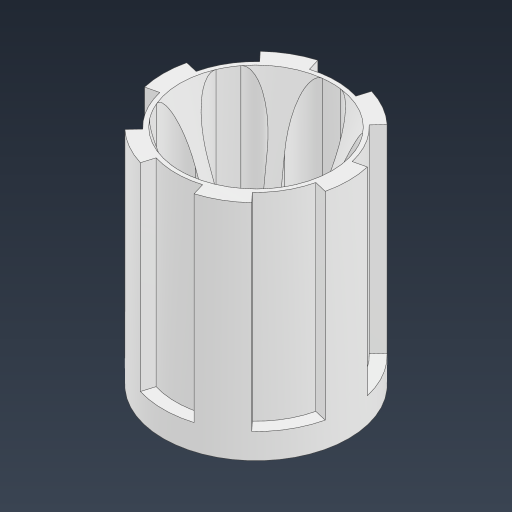
# Autodesk Inventor part: felga
Saved by Autodesk Inventor 2023 (Build 270158000, 158)
## iProperties
Created: 2024-06-08
Part Number: felga
Material: ABS Plastic
Document SubType Name: Modeling
Designer: szymo
Density: 1.06 g/cm^3
Appearance: Smooth - White
Mass: 25.2553 g
Surface Area: 202.96 cm^2
Volume: 23.8257 cm^3
Author: szymo
Autodesk Inventor part; units mm, degrees
ref_plane "YZ Plane" through (0, 0, 0) normal (1, 0, 0) x (0, 1, 0)
ref_plane "XZ Plane" through (0, 0, 0) normal (0, 1, 0) x (-1, 0, 0)
ref_plane "XY Plane" through (0, 0, 0) normal (0, 0, 1) x (1, 0, 0)
sketch "Sketch1" plane through (0, 0, 0) normal (0, 1, 0) x (-1, 0, 0)
  circle A0 centre (0, 0) radius 25
  circle A1 centre (0, 0) radius 22
  circle A2 centre (0, 0) radius 18
  dimension "d0" = 50
  dimension "d1" = 3
  dimension "d2" = 4
  constraints: 3 centre point, 3 coincident
  measures "d0" diameter of A0
  measures "d1" radial gap between concentric circles of A0 A1
  measures "d2" radial gap between concentric circles of A1 A2
extrude "Extrusion1" add sketch "Sketch1" along normal blind 53 contours A1
sketch "Sketch2" plane through (0, 0, 0) normal (0, 1, 0) x (-1, 0, 0)
  circle A0 centre (0, 0) radius 22 projected
  circle A1 centre (0, 0) radius 18 projected
  circle A2 centre (0, 0) radius 5
  line L0 (0, 0) -> (18, 0) construction
  circle A3 centre (0, 0) radius 18 projected
  line L1 (4.7697, 1.5) -> (17.9374, 1.5)
  line L2 (17.9374, -1.5) -> (4.7697, -1.5)
  line L3 (1.0858, 4.8807) -> (7.6697, 16.2842)
  line L4 (0, 0) -> (9, 15.5885) construction
  line L5 (10.2677, 14.7842) -> (3.6839, 3.3807)
  line L6 (-3.6839, 3.3807) -> (-10.2677, 14.7842)
  line L7 (0, 0) -> (-9, 15.5885) construction
  line L8 (-7.6697, 16.2842) -> (-1.0858, 4.8807)
  line L9 (-4.7697, -1.5) -> (-17.9374, -1.5)
  line L10 (0, 0) -> (-18, 0) construction
  line L11 (-17.9374, 1.5) -> (-4.7697, 1.5)
  line L12 (-1.0858, -4.8807) -> (-7.6697, -16.2842)
  line L13 (0, 0) -> (-9, -15.5885) construction
  line L14 (-10.2677, -14.7842) -> (-3.6839, -3.3807)
  line L15 (3.6839, -3.3807) -> (10.2677, -14.7842)
  line L16 (0, 0) -> (9, -15.5885) construction
  line L17 (7.6697, -16.2842) -> (1.0858, -4.8807)
  point P0 (3.6839, 3.3807)
  point P1 (10.2677, 14.7842)
  point P2 (7.6697, 16.2842)
  point P3 (1.0858, 4.8807)
  point P4 (-1.0858, 4.8807)
  point P5 (-7.6697, 16.2842)
  point P6 (-3.6839, 3.3807)
  point P7 (-4.7697, 1.5)
  point P8 (-17.9374, 1.5)
  point P9 (-4.7697, -1.5)
  point P10 (-3.6839, -3.3807)
  point P11 (-10.2677, -14.7842)
  point P12 (-7.6697, -16.2842)
  point P13 (-1.0858, -4.8807)
  point P14 (1.0858, -4.8807)
  point P15 (10.2677, -14.7842)
  point P16 (3.6839, -3.3807)
  dimension "d5" = 10
  dimension "d6" = 1.5
  dimension "d7" = 1.5
  dimension "d10" = 360
  constraints: 36 end point, 5 point on circle, 2 parallel, 1 centre point, 1 coincident, 1 horizontal, 55 other
  measures "d5" diameter of A2
  measures "d6" distance between parallel lines of L1 L0
  measures "d7" distance between parallel lines of L0 L2
extrude "Extrusion2" add sketch "Sketch2" along normal blind 17 contours A1 L2 A2 L1 | L5 A2 L3 A1 | A2 | A1 L17 A2 L15 | L8 A2 L6 A1 | A1 L14 A2 L12 | L11 A2 L9 A1
chamfer "Chamfer1" distance 36 distance2 13 7 edges at (9, 17, 15.5885) (18, 17, 0) (9, 17, -15.5885) (-9, 17, -15.5885) (-17.9843, 17, 0.7507) (-17.9843, 17, -0.7507) (-9, 17, 15.5885) measured on face at (-17.9843, 17.5, 0.7507) measured on face at (-9, 17.5, 15.5885) measured on face at (9, 17.5, 15.5885) measured on face at (-17.9843, 17.5, -0.7507) measured on face at (18, 17.5, 0) measured on face at (9, 17.5, -15.5885) measured on face at (-9, 17.5, -15.5885)
sketch "Sketch3" plane through (0, 0, 0) normal (0, -1, 0) x (1, 0, 0)
  circle A0 centre (0, 0) radius 3
  line L0 (-1.9261, 2.3) -> (1.9261, 2.3)
  line L1 (1.9261, -2.3) -> (-1.9261, -2.3)
  dimension "d19" = 6
  dimension "d20" = 4.6
  dimension "d21" = 2.3
  dimension "d22" = 2.3
  constraints: 4 end point, 4 point on circle, 1 centre point, 1 coincident, 1 horizontal, 1 parallel
  measures "d19" diameter of A0
  measures "d20" distance between parallel lines of L0 L1
  measures "d21" distance from line of L0 point (0, 0)
  measures "d22" distance from line of L1 point (0, 0)
extrude "Extrusion3" cut sketch "Sketch3" against normal blind 12 contours A0 L1 L0
sketch "Sketch6" plane through (0, 0, 0) normal (0, -1, 0) x (1, 0, 0)
  circle A0 centre (0, 0) radius 22 projected
  circle A1 centre (0, -10) radius 3.5
  arc A2 (-7.6697, -16.2842) -> (7.6697, -16.2842) centre (0, 0) ccw projected
  arc A3 (-7.6697, -16.2842) -> (7.6697, -16.2842) centre (0, 0) ccw projected
  circle A4 centre (0, -14.8667) radius 3.1333
  circle A5 centre (12.8749, -7.4333) radius 3.1333
  circle A6 centre (8.6603, -5) radius 3.5
  circle A7 centre (12.8749, 7.4333) radius 3.1333
  circle A8 centre (8.6603, 5) radius 3.5
  circle A9 centre (0, 14.8667) radius 3.1333
  circle A10 centre (0, 10) radius 3.5
  circle A11 centre (-12.8749, 7.4333) radius 3.1333
  circle A12 centre (-8.6603, 5) radius 3.5
  circle A13 centre (-12.8749, -7.4333) radius 3.1333
  circle A14 centre (-8.6603, -5) radius 3.5
  line L0 (-1.0858, -4.8807) -> (-7.6697, -16.2842) projected
  arc A15 (-1.0858, -4.8807) -> (1.0858, -4.8807) centre (0, 0) ccw projected
  line L1 (7.6697, -16.2842) -> (1.0858, -4.8807) projected
  arc A16 (1.0858, 4.8807) -> (-1.0858, 4.8807) centre (0, 0) ccw projected
  arc A17 (4.7697, 1.5) -> (3.6839, 3.3807) centre (0, 0) ccw projected
  arc A18 (3.6839, -3.3807) -> (4.7697, -1.5) centre (0, 0) ccw projected
  arc A19 (-1.0858, -4.8807) -> (1.0858, -4.8807) centre (0, 0) ccw projected
  arc A20 (-4.7697, -1.5) -> (-3.6839, -3.3807) centre (0, 0) ccw projected
  arc A21 (-3.6839, 3.3807) -> (-4.7697, 1.5) centre (0, 0) ccw projected
  line L2 (-1.9261, 2.3) -> (1.9261, 2.3) projected
  arc A22 (1.9261, -2.3) -> (1.9261, 2.3) centre (0, 0) ccw projected
  line L3 (1.9261, -2.3) -> (-1.9261, -2.3) projected
  arc A23 (-1.9261, 2.3) -> (-1.9261, -2.3) centre (0, 0) ccw projected
  arc A24 (-7.6697, -16.2842) -> (7.6697, -16.2842) centre (0, 0) ccw projected
  line L4 (-1.0858, -4.8807) -> (-7.6697, -16.2842) projected
  arc A25 (-1.0858, -4.8807) -> (1.0858, -4.8807) centre (0, 0) ccw projected
  line L5 (7.6697, -16.2842) -> (1.0858, -4.8807) projected
  line L6 (3.6839, -3.3807) -> (10.2677, -14.7842) projected
  arc A26 (3.6839, -3.3807) -> (4.7697, -1.5) centre (0, 0) ccw projected
  line L7 (17.9374, -1.5) -> (4.7697, -1.5) projected
  arc A27 (10.2677, -14.7842) -> (17.9374, -1.5) centre (0, 0) ccw projected
  line L8 (4.7697, 1.5) -> (17.9374, 1.5) projected
  arc A28 (4.7697, 1.5) -> (3.6839, 3.3807) centre (0, 0) ccw projected
  line L9 (10.2677, 14.7842) -> (3.6839, 3.3807) projected
  arc A29 (17.9374, 1.5) -> (10.2677, 14.7842) centre (0, 0) ccw projected
  line L10 (1.0858, 4.8807) -> (7.6697, 16.2842) projected
  arc A30 (1.0858, 4.8807) -> (-1.0858, 4.8807) centre (0, 0) ccw projected
  line L11 (-7.6697, 16.2842) -> (-1.0858, 4.8807) projected
  arc A31 (7.6697, 16.2842) -> (-7.6697, 16.2842) centre (0, 0) ccw projected
  line L12 (-3.6839, 3.3807) -> (-10.2677, 14.7842) projected
  arc A32 (-3.6839, 3.3807) -> (-4.7697, 1.5) centre (0, 0) ccw projected
  line L13 (-17.9374, 1.5) -> (-4.7697, 1.5) projected
  arc A33 (-10.2677, 14.7842) -> (-17.9374, 1.5) centre (0, 0) ccw projected
  circle A34 centre (0, 0) radius 22 projected
  line L14 (-4.7697, -1.5) -> (-17.9374, -1.5) projected
  arc A35 (-4.7697, -1.5) -> (-3.6839, -3.3807) centre (0, 0) ccw projected
  line L15 (-10.2677, -14.7842) -> (-3.6839, -3.3807) projected
  arc A36 (-17.9374, -1.5) -> (-10.2677, -14.7842) centre (0, 0) ccw projected
  arc A37 (-1.0858, 4.8807) -> (-3.6839, 3.3807) centre (0, 0) ccw projected
  arc A38 (3.6839, 3.3807) -> (1.0858, 4.8807) centre (0, 0) ccw projected
  arc A39 (4.7697, -1.5) -> (4.7697, 1.5) centre (0, 0) ccw projected
  arc A40 (1.0858, -4.8807) -> (3.6839, -3.3807) centre (0, 0) ccw projected
  arc A41 (-3.6839, -3.3807) -> (-1.0858, -4.8807) centre (0, 0) ccw projected
  arc A42 (-4.7697, 1.5) -> (-4.7697, -1.5) centre (0, 0) ccw projected
  point P0 (0, -18)
  point P1 (3.0311, -8.25)
  point P2 (-3.0311, -8.25)
  point P3 (8.6603, -1.5)
  point P4 (4.7697, -1.5)
  point P5 (3.6839, -3.3807)
  point P6 (5.6292, -6.75)
  point P7 (5.6292, 6.75)
  point P8 (3.6839, 3.3807)
  point P9 (4.7697, 1.5)
  point P10 (8.6603, 1.5)
  point P11 (-3.0311, 8.25)
  point P12 (-1.0858, 4.8807)
  point P13 (1.0858, 4.8807)
  point P14 (3.0311, 8.25)
  point P15 (-8.6603, 1.5)
  point P16 (-4.7697, 1.5)
  point P17 (-3.6839, 3.3807)
  point P18 (-5.6292, 6.75)
  point P19 (-5.6292, -6.75)
  point P20 (-3.6839, -3.3807)
  point P21 (-4.7697, -1.5)
  point P22 (-8.6603, -1.5)
  dimension "d40" = 7
  dimension "d51" = 360
  constraints: 12 centre point, 1 tangent, 25 other
  measures "d40" diameter of A1
extrude "fillleeciki" add sketch "Sketch6" against normal up to surface contours A1 L0 A15 L1 | A18 L7 A6 L6 | L15 A14 L14 A20 | A17 L9 A8 L8 | L13 A12 L12 A21 | A16 L11 A10 L10 round surface about axis through (0, 35, 0) along (0, 1, 0) radius 11.5 half angle 19.855214 far side no
sketch "Sketch5" plane through (0, 17, 0) normal (0, 1, 0) x (1, 0, 0)
  point P0 (0, 0)
  point P1 (0, 0)
  constraints: 1 coincident
hole "Hole2" at (0, 17, 0) direction (0, -1, 0) diameter 3.6 end through all counterbore diameter 6.5 counterbore depth 0 clearance for "Slotted Cheese Head Screw ISO 1207" size "M3" standard "ISO"
ref_plane "Work Plane2" through (0, 53, 0) normal (0, 1, 0) x (1, 0, 0)
sketch "Sketch8" plane through (0, 53, 0) normal (0, 1, 0) x (1, 0, 0)
  line L0 (0, 0) -> (-24.2406, -13.9953) construction
  line L1 (0, 0) -> (-23.7201, 13.6948) construction
  line L2 (0, 0) -> (-9.1053, 0) construction
  arc A0 (-17.9374, -1.5) -> (-10.2677, -14.7842) centre (0, 0) ccw projected
  circle A1 centre (0, 0) radius 22 projected
  circle A2 centre (0, 0) radius 1.8 projected
  circle A3 centre (0, 0) radius 19
  line L3 (-18.5028, -4.3182) -> (-21.4243, -5)
  circle A4 centre (0, 0) radius 22 projected
  line L4 (-18.5028, 4.3182) -> (-21.4243, 5)
  line L5 (-5.5117, -18.183) -> (-6.382, -21.054)
  line L6 (-12.9911, -13.8648) -> (-15.0423, -16.054)
  circle A5 centre (0, 0) radius 19
  line L7 (12.9911, -13.8648) -> (15.0423, -16.054)
  line L8 (5.5117, -18.183) -> (6.382, -21.054)
  circle A6 centre (0, 0) radius 19
  line L9 (18.5028, 4.3182) -> (21.4243, 5)
  line L10 (18.5028, -4.3182) -> (21.4243, -5)
  circle A7 centre (0, 0) radius 19
  line L11 (5.5117, 18.183) -> (6.382, 21.054)
  line L12 (12.9911, 13.8648) -> (15.0423, 16.054)
  circle A8 centre (0, 0) radius 19
  line L13 (-12.9911, 13.8648) -> (-15.0423, 16.054)
  line L14 (-5.5117, 18.183) -> (-6.382, 21.054)
  circle A9 centre (0, 0) radius 19
  point P0 (5.5117, -18.183)
  point P1 (-5.5117, -18.183)
  point P2 (-6.382, -21.054)
  point P3 (21.4243, -5)
  point P4 (18.5028, -4.3182)
  point P5 (12.9911, -13.8648)
  point P6 (15.0423, 16.054)
  point P7 (12.9911, 13.8648)
  point P8 (21.4243, 5)
  point P9 (-6.382, 21.054)
  point P10 (5.5117, 18.183)
  point P11 (6.382, 21.054)
  point P12 (-12.9911, 13.8648)
  point P13 (-15.0423, 16.054)
  point P14 (-21.4243, 5)
  point P15 (-15.0423, -16.054)
  point P16 (-12.9911, -13.8648)
  point P17 (-21.4243, -5)
  dimension "d59" = 30
  dimension "d60" = 30
  dimension "d61" = 1
  dimension "d66" = 5
  dimension "d67" = 5
  dimension "d70" = 360
  constraints: 30 end point, 14 point on circle, 6 centre point, 2 coincident, 2 line through centre, 1 horizontal, 49 other
  measures "d59" angle of L2 L1
  measures "d60" angle of L0 L2
  measures "d61" radial gap between concentric circles of A3 A0
  measures "d66" distance from line of L3.end L2
  measures "d67" vertical distance of L4.end L2.end
extrude "Extrusion5" cut sketch "Sketch8" against normal blind 47 contours L9 A3 L12 A1 | A1 L7 A3 L10 | L11 A3 L14 A1 | A1 L5 A3 L8 | L13 A3 L4 A1 | A1 L3 A3 L6
fillet "Fillet4" radius 4 12 edges at (-7.6697, 26.4999, -16.2842) (7.6697, 26.4999, -16.2842) (10.2677, 26.4999, -14.7842) (17.9374, 26.4999, -1.5) (17.9374, 26.4999, 1.5) (10.2677, 26.4999, 14.7842) (7.6697, 26.4999, 16.2842) (-10.2677, 26.4999, 14.7842) (-7.6697, 26.4999, 16.2842) (-17.9374, 26.4999, -1.5) (-17.9374, 26.4999, 1.5) (-10.2677, 26.4999, -14.7842)
fillet "Fillet6" radius 1 4 edges at (3, 0, 0) (0, 0, -2.3) (0, 0, 2.3) (-3, 0, 0)
equation "\"d7\" = d6"
equation "\"d21\" = d22"
body "Solid1"
